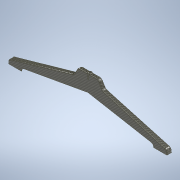
# Autodesk Inventor part: ramynko
Saved by Autodesk Inventor 2022 (Build 260153000, 153)
## iProperties
Created: 2021-05-18
Part Number: ramynko
Material: Všeobecné
Document SubType Name: Modeling
Designer: peepu
Density: 1 g/cm^3
Appearance: Uhlíkové vlákno 1
Author: peepu
Autodesk Inventor part; units mm, degrees
ref_plane "YZ Plane" through (0, 0, 0) normal (1, 0, 0) x (0, 1, 0)
ref_plane "XZ Plane" through (0, 0, 0) normal (0, 1, 0) x (-1, 0, 0)
ref_plane "XY Plane" through (0, 0, 0) normal (0, 0, 1) x (1, 0, 0)
sketch "Náčrt1" plane through (0, 0, 0) normal (0, 0, 1) x (1, 0, 0)
  line L0 (0, 92) -> (25, 92)
  arc A0 (33.7614, 86.8206) -> (25, 92) centre (25, 82) ccw
  line L1 (33.7614, 86.8206) -> (41.2386, 73.2308)
  arc A1 (41.2386, 73.2308) -> (47.2134, 68.4475) centre (50, 78.0514) ccw
  line L2 (47.2134, 68.4475) -> (232.7866, 14.6039)
  arc A2 (240, 5) -> (232.7866, 14.6039) centre (230, 5) ccw
  line L3 (240, 5) -> (240, 0)
  line L4 (240, 0) -> (200, 0)
  arc A3 (200, 0) -> (191.7365, 9.8481) centre (190, 0) ccw
  line L5 (191.7365, 9.8481) -> (0, 43.6564)
  line L6 (0, 43.6564) -> (0, 92)
  point P0 (0, 0)
  dimension "d0" = 10
  dimension "d1" = 92
  dimension "d2" = 240
  dimension "d3" = 0
  dimension "d4" = 10
  dimension "d5" = 0
  dimension "d6" = 10
  dimension "d7" = 10
  dimension "d8" = 40
  dimension "d9" = 50
  dimension "d10" = 25
  dimension "d12" = 10
  dimension "d13" = 135
  dimension "d16" = 5
  constraints: 14 end point, 8 point on circle, 7 tangent, 4 centre point, 2 horizontal, 2 vertical
  measures "d0" radius of A0
  measures "d1" distance of point (0, 0) L0.start
  measures "d2" distance of L3.end point (0, 0)
  measures "d3" distance from line of point (0, 0) L4
  measures "d4" radius of A3
  measures "d5" distance from line of point (0, 0) L6
  measures "d6" radius of A1
  measures "d7" radius of A2
  measures "d8" distance of L3.end L4.end
  measures "d9" horizontal distance of A1.centre L0.start
  measures "d10" horizontal distance of L0.start A0.centre
  measures "d12" angle of L0 L5
  measures "d13" angle of L2 L1
  measures "d16" distance from line of L4 L3.start
sketch "Náčrt2" plane through (0, 0, 0) normal (0, 1, 0) x (-1, 0, 0)
  line L0 (240, 7.5) -> (-240, 7.5)
  line L1 (-240, 7.5) -> (-240, -7.5)
  line L2 (-240, -7.5) -> (240, -7.5)
  line L3 (240, -7.5) -> (240, 7.5)
  line L4 (240, 7.5) -> (-240, -7.5) construction
  line L5 (-240, 7.5) -> (240, -7.5) construction
  point P0 (0, 0)
  dimension "d14" = 480
  dimension "d15" = 15
  constraints: 12 end point, 2 midpoint, 2 parallel, 1 horizontal, 1 perpendicular
  measures "d14" distance of L2.end L1.end
  measures "d15" distance of L1.end L0.end
extrude "Vysunutí1" add sketch "Náčrt2" along normal blind 92 draft -1.5
extrude "Vysunutí2" cut sketch "Náčrt1" along normal mid plane 20 keep common part
mirror "Zrcadlit1" about plane through (0, 92, 0) normal (-1, 0, 0)
fillet "Zaoblení1" radius 2 26 edges at (-237.3892, 11.7379, 7.1926) (-43.7503, 70.2449, 5.6606) (-37.5, 80.0257, 5.4045) (-30.0889, 90.6083, 5.1273) (0, 92, 5.0909) (30.0889, 90.6083, 5.1273) (37.5, 80.0257, 5.4045) (43.7503, 70.2449, 5.6606) (140, 41.5257, 6.4126) (237.3892, 11.7379, 7.1926) (-140, 41.5257, 6.4126) (30.0889, 90.6083, -5.1273) (37.5, 80.0257, -5.4045) (43.7503, 70.2449, -5.6606) (140, 41.5257, -6.4126) (237.3892, 11.7379, -7.1926) (-30.0889, 90.6083, -5.1273) (-37.5, 80.0257, -5.4045) (-43.7503, 70.2449, -5.6606) (-140, 41.5257, -6.4126) (-237.3892, 11.7379, -7.1926) (0, 92, -5.0909) (239.9098, 3.4456, 7.4098) (239.9098, 3.4456, -7.4098) (-239.9098, 3.4456, -7.4098) (-239.9098, 3.4456, 7.4098)
shell "Skořepina1" thickness 1 removed faces 6 at (-225.3338, 0, -2.5) at (-127.8243, 21.1175, -2.1189) at (-199.927, 1.2064, -2.4928) at (225.3338, 0, 2.5) at (199.927, 1.2064, -2.4928) at (127.8243, 21.1175, -2.1189)
sketch "Náčrt4" plane through (0, 0, 0) normal (0, 0, 1) x (1, 0, 0)
  line L0 (0, 94) -> (5.5, 94)
  line L1 (5.5, 94) -> (5.5, 54)
  line L2 (5.5, 54) -> (0, 54)
  line L3 (0, 54) -> (0, 94)
  line L4 (25, 92) -> (-25, 92) projected
  line L5 (-95.7716, 245.2696) -> (88.1139, 245.2696) construction
  line L6 (88.1139, 245.2696) -> (88.1139, 107.4217) construction
  line L7 (88.1139, 107.4217) -> (-95.7716, 107.4217) construction
  line L8 (-95.7716, 107.4217) -> (-95.7716, 245.2696) construction
  point P0 (0, 0)
  dimension "d23" = 5.5
  dimension "d24" = 40
  dimension "d25" = 2
  constraints: 8 end point, 2 parallel, 1 horizontal, 1 perpendicular, 2 other
  measures "d23" distance of L1.end L2.end
  measures "d24" distance of L0.end L1.end
  measures "d25" distance between parallel lines of L4 L0
revolve "Rotace1" add sketch "Náčrt4" angle 360 about axis through (0, 54, 0) along (0, 1, 0)
fillet "Zaoblení2" radius 2 1 edges at (-5.5, 94, 0)
sketch "Náčrt5" plane through (0, 94, 0) normal (0, 1, 0) x (1, 0, 0)
  point P0 (0, 0)
  point P1 (0, 0)
  constraints: 1 coincident
hole "Díra1" at (0, 94, 0) direction (0, -1, 0) diameter 6 end through all
